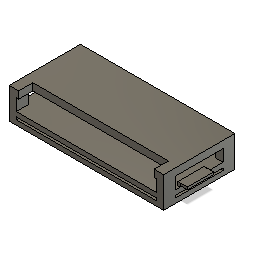
DryFoodDispenser (Autodesk Fusion 360 archive; units mm, degrees)
design "RPi_w_heatsink"
Autodesk Fusion 360 part; units mm, degrees
note: some values were not read from the file. Chosen so that the rebuilt part matches the saved one: which bodies a step acts on.
sketch "Sketch1" plane through (0, 0, 0) normal (0, 1, 0) x (1, 0, 0)
  line L0 (-30, 10) -> (35, 10)
  line L1 (35, 10) -> (35, -20)
  line L2 (35, -20) -> (-30, -20)
  line L3 (-30, -20) -> (-30, 10)
  dimension "d1" = 65
  dimension "d2" = 30
  constraint horizontal L0
  constraint vertical L1
  constraint horizontal L2
  constraint vertical L3
  measures "d1" distance of L0.start L0.end
  measures "d2" distance of L0.start L2.end
extrude "Extrude1" add sketch "Sketch1" along normal blind 13 makes body 1
sketch "Sketch2" plane through (0, 0, -10) normal (0, 0, -1) x (-1, 0, 0)
  line L0 (-35, 0) -> (30, 0)
  line L1 (30, 0) -> (30, 13)
  line L2 (30, 13) -> (-35, 13)
  line L3 (-35, 13) -> (-35, 0)
  line L4 (-32, 3) -> (27, 3)
  line L5 (27, 3) -> (27, 2)
  line L6 (27, 2) -> (-32, 2)
  line L7 (-32, 2) -> (-32, 3)
  dimension "d5" = 59
  dimension "d6" = 1
  constraint horizontal L4
  constraint vertical L5
  constraint horizontal L6
  constraint vertical L7
  measures "d5" distance of L4.start L4.end
  measures "d6" distance of L4.start L6.end
sketch "Sketch3" plane through (0, 0, -10) normal (0, 0, -1) x (-1, 0, 0)
  line L0 (-32, 10) -> (27, 10)
  line L1 (27, 10) -> (27, 5)
  line L2 (27, 5) -> (-32, 5)
  line L3 (-32, 5) -> (-32, 10)
  dimension "d7" = 59
  dimension "d8" = 5
  constraint horizontal L0
  constraint vertical L1
  constraint horizontal L2
  constraint vertical L3
  measures "d7" distance of L0.start L0.end
  measures "d8" distance of L0.start L2.end
extrude "Extrude2" cut sketch "Sketch2" sketch "Sketch3" against normal blind 32 contours L4 L5 L6 L7 of sketch 2 bodies 1
sketch "Sketch4" plane through (35, 0, 0) normal (1, 0, 0) x (0, 0, -1)
  line L0 (-20, 0) -> (10, 0)
  line L1 (10, 0) -> (10, 13)
  line L2 (10, 13) -> (-20, 13)
  line L3 (-20, 13) -> (-20, 0)
  line L4 (-15, 10) -> (5, 10)
  line L5 (5, 10) -> (5, 5)
  line L6 (5, 5) -> (-15, 5)
  line L7 (-15, 5) -> (-15, 10)
  line L8 (-15, 3) -> (5, 3)
  line L9 (5, 3) -> (5, 2)
  line L10 (5, 2) -> (-15, 2)
  line L11 (-15, 2) -> (-15, 3)
  dimension "d11" = 20
  dimension "d12" = 5
  dimension "d13" = 20
  dimension "d14" = 1
  constraint horizontal L4
  constraint vertical L5
  constraint horizontal L6
  constraint vertical L7
  constraint horizontal L8
  constraint vertical L9
  constraint horizontal L10
  constraint vertical L11
  measures "d11" distance of L4.start L4.end
  measures "d12" distance of L4.start L6.end
  measures "d13" distance of L8.start L8.end
  measures "d14" distance of L8.start L10.end
extrude "Extrude3" cut sketch "Sketch4" against normal blind 79 contours L4 L5 L6 L7 | L8 L9 L10 L11 bodies 1
sketch "Sketch5" plane through (0, 0, 0) normal (0, 0, 1) x (1, 0, 0)
  line L0 (29.5, 9, -10) -> (16.5, 9, -10)
  line L1 (16.5, 9, -10) -> (16.5, 5, -10)
  line L2 (16.5, 5, -10) -> (29.5, 5, -10)
  line L3 (29.5, 5, -10) -> (29.5, 9, -10)
  line L4 (-1.5, 8, -10) -> (-9.5, 8, -10)
  line L5 (-9.5, 8, -10) -> (-9.5, 5, -10)
  line L6 (-9.5, 5, -10) -> (-1.5, 5, -10)
  line L7 (-1.5, 5, -10) -> (-1.5, 8, -10)
  line L8 (-15, 8, -10) -> (-23, 8, -10)
  line L9 (-23, 8, -10) -> (-23, 5, -10)
  line L10 (-23, 5, -10) -> (-15, 5, -10)
  line L11 (-15, 5, -10) -> (-15, 8, -10)
  dimension "d17" = 13
  dimension "d18" = 4
  dimension "d19" = 8
  dimension "d20" = 3
  dimension "d21" = 8
  dimension "d22" = 3
sketch "Sketch5 (curves -10 mm off its plane)" plane through (0, 0, -10) normal (0, 0, 1) x (1, 0, 0)
  line L0 (29.5, 9) -> (16.5, 9)
  line L1 (16.5, 9) -> (16.5, 5)
  line L2 (16.5, 5) -> (29.5, 5)
  line L3 (29.5, 5) -> (29.5, 9)
  line L4 (-1.5, 8) -> (-9.5, 8)
  line L5 (-9.5, 8) -> (-9.5, 5)
  line L6 (-9.5, 5) -> (-1.5, 5)
  line L7 (-1.5, 5) -> (-1.5, 8)
  line L8 (-15, 8) -> (-23, 8)
  line L9 (-23, 8) -> (-23, 5)
  line L10 (-23, 5) -> (-15, 5)
  line L11 (-15, 5) -> (-15, 8)
extrude "Extrude4" add sketch "Sketch5 (curves -10 mm off its plane)" against normal blind 2 contours L4 L5 L6 L7 | L8 L9 L10 L11 bodies 1
extrude "Extrude5" add sketch "Sketch5 (curves -10 mm off its plane)" against normal blind 1 contours L0 L1 L2 L3 bodies 1
sketch "Sketch6" plane through (0, 0, 0) normal (1, 0, 0) x (0, 0, -1)
  line L0 (-13, 6.5, 35) -> (-2, 6.5, 35)
  line L1 (-2, 6.5, 35) -> (-2, 5.5, 35)
  line L2 (-2, 5.5, 35) -> (-13, 5.5, 35)
  line L3 (-13, 5.5, 35) -> (-13, 6.5, 35)
  dimension "d27" = 11
  dimension "d28" = 1
sketch "Sketch6 (curves 35 mm off its plane)" plane through (35, 0, 0) normal (1, 0, 0) x (0, 0, -1)
  line L0 (-13, 6.5) -> (-2, 6.5)
  line L1 (-2, 6.5) -> (-2, 5.5)
  line L2 (-2, 5.5) -> (-13, 5.5)
  line L3 (-13, 5.5) -> (-13, 6.5)
extrude "Extrude6" add sketch "Sketch6 (curves 35 mm off its plane)" along normal blind 3 separate body makes body 2
combine "Combine1" operation add target body 1 tool bodies 2 makes body 3 at (36, 6.5, 9.3333)
combine "Combine2" operation add target body 1 tool bodies 3 makes body 4 at (36, 6.5, 9.3333)
sketch "Sketch7" plane through (0, 5, 0) normal (0, 1, 0) x (-1, 0, 0)
  line L0 (27, 15) -> (27, 20)
  line L1 (27, 20) -> (-32, 20)
  line L2 (-32, 20) -> (-32, 15)
  line L3 (-32, 15) -> (-35, 15)
  line L4 (-35, 15) -> (-35, -5)
  line L5 (-35, -5) -> (-32, -5)
  line L6 (-32, -5) -> (-32, -10)
  line L7 (-32, -10) -> (-29.5, -10)
  line L8 (-29.5, -10) -> (-16.5, -10)
  line L9 (-16.5, -10) -> (1.5, -10)
  line L10 (1.5, -10) -> (9.5, -10)
  line L11 (9.5, -10) -> (15, -10)
  line L12 (15, -10) -> (23, -10)
  line L13 (23, -10) -> (27, -10)
  line L14 (27, -10) -> (27, -5)
  line L15 (27, -5) -> (30, -5)
  line L16 (30, -5) -> (30, 15)
  line L17 (30, 15) -> (27, 15)
  line L18 (-35, 13.0223) -> (-34, 13.0223)
  line L19 (-34, 13.0223) -> (-34, 2.0223)
  line L20 (-34, 2.0223) -> (-35, 2.0223)
  line L21 (-35, 2.0223) -> (-35, 13.0223)
  dimension "d31" = 1
  dimension "d32" = 11
  constraint horizontal L18
  constraint vertical L19
  constraint horizontal L20
  constraint vertical L21
  constraint coincident L4 L18.start
  measures "d31" distance of L18.start L18.end
  measures "d32" distance of L18.start L20.end
extrude "Extrude7" add sketch "Sketch7" along normal blind 1.5 contours L4 L18 L19 L20 L21 bodies 1 4
sketch "Sketch8" plane through (0, 13, 0) normal (0, 1, 0) x (-1, 0, 0)
  line L0 (30, 20) -> (-35, 20)
  line L1 (-35, 20) -> (-35, -10)
  line L2 (-35, -10) -> (30, -10)
  line L3 (30, -10) -> (30, 20)
  line L4 (-31, 20) -> (26, 20)
  line L5 (26, 20) -> (26, 14)
  line L6 (26, 14) -> (-31, 14)
  line L7 (-31, 14) -> (-31, 20)
  dimension "d35" = 57
  dimension "d36" = 6
  constraint horizontal L4
  constraint vertical L5
  constraint horizontal L6
  constraint vertical L7
  measures "d35" distance of L4.start L4.end
  measures "d36" distance of L4.start L6.end
extrude "Extrude8" cut sketch "Sketch8" against normal blind 5 contours L0 L4 L5 L6 L7 bodies 1
